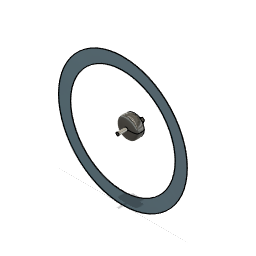
X8_7inch (Autodesk Fusion 360 archive; units mm, degrees)
design "EMAX ECO2 2807"
Autodesk Fusion 360 part; units mm, degrees
sketch "Skizze1" plane through (0, 0, 0) normal (0, 0, 1) x (1, 0, 0)
  circle A0 centre (0, 0) radius 9.5 construction
  line L0 (-6.7175, 6.7175) -> (6.7175, 6.7175) construction
  line L1 (6.7175, 6.7175) -> (6.7175, -6.7175) construction
  line L2 (6.7175, -6.7175) -> (-6.7175, -6.7175) construction
  line L3 (-6.7175, -6.7175) -> (-6.7175, 6.7175) construction
  line L4 (-6.7175, 6.7175) -> (6.7175, -6.7175) construction
  line L5 (6.7175, 6.7175) -> (-6.7175, -6.7175) construction
  circle A1 centre (-6.7175, 6.7175) radius 1.5
  circle A2 centre (6.7175, 6.7175) radius 1.5
  circle A3 centre (6.7175, -6.7175) radius 1.5
  circle A4 centre (-6.7175, -6.7175) radius 1.5
  circle A5 centre (0, 0) radius 17.5 construction
  line L6 (0, 17.5) -> (0, -17.5) construction
  line L7 (17.5, 0) -> (-17.5, 0) construction
  arc A6 (-9.5831, 14.6429) -> (9.5831, 14.6429) centre (0, 17.5) ccw
  arc A7 (14.6429, 9.5831) -> (14.6429, -9.5831) centre (17.5, 0) ccw
  arc A8 (9.5831, -14.6429) -> (-9.5831, -14.6429) centre (0, -17.5) ccw
  arc A9 (10.0071, 6.6225) -> (6.6225, 10.0071) centre (0, 0) ccw
  arc A10 (-14.6429, -9.5831) -> (-14.6429, 9.5831) centre (-17.5, 0) ccw
  arc A11 (-6.6225, 10.0071) -> (-10.0071, 6.6225) centre (0, 0) ccw
  arc A12 (-10.0071, -6.6225) -> (-6.6225, -10.0071) centre (0, 0) ccw
  arc A13 (6.6225, -10.0071) -> (10.0071, -6.6225) centre (0, 0) ccw
  circle A14 centre (0, 0) radius 5
  dimension "d1" = 19
  dimension "d2" = 3
  dimension "d3" = 35
  dimension "d4" = 20
  dimension "d5" = 10
  dimension "d6" = 12
  constraint coincident A0.centre A5.centre
  constraint horizontal L0
  constraint perpendicular L0 L1
  constraint parallel L0 L2
  constraint parallel L1 L3
  constraint coincident A0 L0.start
  constraint coincident L4 A0.centre
  constraint coincident L5 A0.centre
  constraint equal L0 L3
  constraint coincident L0.start L3.end
  constraint coincident L0.end L1.start
  constraint coincident L1.end L2.start
  constraint coincident L2.end L3.start
  constraint equal A1 A2
  constraint equal A1 A4
  constraint equal A2 A3
  constraint concentric A5 A11
  constraint coincident A5 L6.start
  constraint coincident A5 L6.end
  constraint vertical L6
  constraint coincident A5 L7.start
  constraint coincident A5 L7.end
  constraint coincident A0.centre L6
  constraint coincident A0.centre L7
  constraint horizontal L7
  constraint coincident L6.start A6.centre
  constraint coincident L7.start A7.centre
  constraint coincident L6.end A8.centre
  constraint coincident L7.end A10.centre
  constraint equal A6 A10
  constraint equal A6 A7
  constraint equal A7 A8
  constraint coincident A9.end A6
  constraint coincident A11.start A6
  constraint coincident A5 A6.end
  constraint coincident A5 A6.start
  constraint coincident A5 A7.end
  constraint coincident A5 A7.start
  constraint coincident A5 A8.end
  constraint coincident A5 A8.start
  constraint coincident A7 A13.end
  constraint concentric A9 A11
  constraint coincident A7 A9.start
  constraint coincident A5 A10.end
  constraint coincident A5 A10.start
  constraint coincident A10 A12.start
  constraint concentric A11 A12
  constraint coincident A10 A11.end
  constraint coincident A8 A12.end
  constraint concentric A12 A13
  constraint coincident A8 A13.start
  constraint equal A9 A11
  constraint equal A9 A13
  constraint equal A9 A12
  measures "d1" diameter of A0
  measures "d2" diameter of A1
  measures "d3" diameter of A5
  measures "d4" diameter of A6
  measures "d5" diameter of A14
  measures "d6" radius of A9
extrude "Extrusion1" add sketch "Skizze1" along normal blind 6.6 makes body 1
sketch "Skizze3" plane through (0, 0, 0) normal (0, 1, 0) x (1, 0, 0)
  line L0 (-5.2175, -6.6) -> (-8.2175, -6.6)
  line L1 (5, -6.6) -> (-5, -6.6)
  line L2 (-5.2175, -6.6) -> (-8.2175, -6.6)
  line L3 (8.2175, -6.6) -> (5.2175, -6.6)
  line L4 (8.2175, -6.6) -> (5.2175, -6.6)
  line L5 (-10.0071, -6.6) -> (-6.6225, -6.6)
  line L6 (6.6225, -6.6) -> (-6.6225, -6.6)
  line L7 (6.6225, -6.6) -> (10.0071, -6.6)
  line L8 (10.0071, -6.6) -> (7.5, -6.6)
  line L9 (6.6225, -6.6) -> (10.0071, -6.6)
  line L10 (6.6225, -6.6) -> (-6.6225, -6.6)
  line L11 (-10.0071, -6.6) -> (-6.6225, -6.6)
  line L12 (-7.5, -6.6) -> (-10.0071, -6.6)
  line L13 (0, -6.6) -> (16, -6.6)
  spline S0 degree 5 poles (16, -6.6) (16.0942, -6.8538) (16.2705, -7.3729) (16.4989, -8.1862) (16.7304, -9.3406) (16.9005, -10.8897) (16.9635, -12.5072) (16.9487, -14.1142) (16.9133, -15.5669) (16.7566, -16.8027) (16.327, -17.7989) (15.4656, -18.5655) (14.0873, -19.1268) (12.1784, -19.5153) (9.7678, -19.7663) (6.9097, -19.9143) (4.3131, -19.9741) (2.2133, -19.9953) (0.7486, -20) (0, -20) knots 0 0 0 0 0 0 0.066667 0.133333 0.2 0.266667 0.333333 0.4 0.466667 0.533333 0.6 0.666667 0.733333 0.8 0.866667 0.933333 1 1 1 1 1 1
  line L14 (0, -20) -> (0, -6.6)
  line L15 (4.1146, -20) -> (-4.1146, -20)
  line L16 (16.95, -10.2) -> (16.95, -16.2)
  point P0 (16.95, -13.2)
  point P1 (16, -18)
  dimension "d12" = 16.95
  dimension "d13" = 13.4
  dimension "d18" = 6.6
  dimension "d19" = 16
  dimension "d20" = 2
  constraint midpoint L10 L13.start
  constraint parallel L3 L13
  constraint perpendicular L1 L14
  constraint midpoint S0.end L15
  constraint horizontal L15
  constraint midpoint P0 L16
  constraint vertical L16
  constraint vertical L13.end P1
  measures "d12" distance of L14 L16
  measures "d13" distance of L13.start S0.end
  measures "d18" distance of L13 P0
  measures "d19" distance of L13.start L13.end
  measures "d20" distance of P1 S0.end
revolve "Drehen1" add sketch "Skizze3" angle 360 about axis through (0, 0, 20) along (0, 0, -1) bodies 1
sketch "Skizze4" plane through (0, 0, 6.6) normal (0, 0, -1) x (-1, 0, 0)
  circle A0 centre (0, 0) radius 5
  circle A1 centre (0, 0) radius 2.5
  dimension "d15" = 5
  constraint coincident A0.centre A1.centre
  measures "d15" diameter of A1
extrude "Extrusion3" add sketch "Skizze4" against normal blind 27.5 contours A1 bodies 1
ref_plane "Arbeitsebene1" through (0, 0, 25.1) normal (0, 0, 1) x (1, 0, 0)
sketch "Skizze6" plane through (0, 0, 25.1) normal (0, 0, 1) x (1, 0, 0)
  circle A0 centre (0, 0) radius 85.4
  circle A1 centre (0, 0) radius 105
  dimension "d22" = 210
  dimension "d23" = 170.8
  constraint coincident A0.centre A1.centre
  constraint concentric A0 A1
  measures "d22" diameter of A1
  measures "d23" diameter of A0
extrude "Extrusion5" add sketch "Skizze6" along normal blind 0.5 separate body makes body 2
equation "d12 = ( 33.9 / 2 ) * 1 mm"
